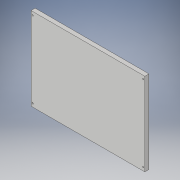
# Autodesk Inventor part: espHolder
Saved by Autodesk Inventor 2019.4 (Build 234330000, 330)
## iProperties
Created: 2019-10-23
Part Number: espHolder
Material: Generic
Document SubType Name: Modeling
Designer: nLaptop
Density: 1 g/cm^3
Appearance: Default
Author: nLaptop
Autodesk Inventor part; units mm, degrees
ref_plane "YZ Plane" through (0, 0, 0) normal (1, 0, 0) x (0, 1, 0)
ref_plane "XZ Plane" through (0, 0, 0) normal (0, 1, 0) x (-1, 0, 0)
ref_plane "XY Plane" through (0, 0, 0) normal (0, 0, 1) x (1, 0, 0)
sketch "Sketch1" plane through (0, 0, 0) normal (0, 0, 1) x (1, 0, 0)
  line L0 (0, 25.4) -> (-34.925, 25.4)
  line L1 (-34.925, 25.4) -> (-34.925, 0)
  line L2 (-34.925, 0) -> (-34.925, -25.4)
  line L3 (-34.925, -25.4) -> (34.925, -25.4)
  line L4 (34.925, -25.4) -> (34.925, 25.4)
  line L5 (34.925, 25.4) -> (0, 25.4)
  line L6 (34.925, 25.4) -> (34.925, 23.368)
  line L7 (-34.925, 25.4) -> (-34.925, 23.368)
  circle A0 centre (33.909, -23.368) radius 0.4064
  circle A1 centre (33.909, 23.368) radius 0.4064
  circle A2 centre (-33.909, 23.368) radius 0.4064
  circle A3 centre (-33.909, -23.368) radius 0.4064
  point P0 (0, 0)
  dimension "d11" = 0.8128
  dimension "d12" = 0.8128
  dimension "d13" = 0.8128
  dimension "d14" = 0.8128
  constraints: 16 end point, 4 centre point, 4 perpendicular, 4 point on line
  measures "d11" diameter of A0
  measures "d12" diameter of A1
  measures "d13" diameter of A2
  measures "d14" diameter of A3
extrude "Extrusion1" add sketch "Sketch1" along normal blind 2.54
body "Solid1"
